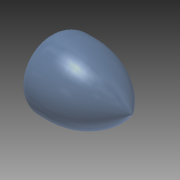
# Autodesk Inventor part: eye
Saved by Autodesk Inventor 2015 (Build 190159000, 159)
## iProperties
Created: 2015-03-17
Part Number: eye
Material: Genérico
Document SubType Name: Modeling
Designer: david_000
Density: 1 g/cm^3
Appearance: Valor por defecto
Author: david_000
Autodesk Inventor part; units mm, degrees
ref_plane "YZ Plane" through (0, 0, 0) normal (1, 0, 0) x (0, 1, 0)
ref_plane "XZ Plane" through (0, 0, 0) normal (0, 1, 0) x (-1, 0, 0)
ref_plane "XY Plane" through (0, 0, 0) normal (0, 0, 1) x (1, 0, 0)
sketch "Boceto1" plane through (0, 0, 0) normal (0, 1, 0) x (-1, 0, 0)
  line L0 (135, 0) -> (135, 20)
  line L1 (135, 20) -> (135, 65)
  line L2 (135, 65) -> (35, 65)
  line L3 (135, 0) -> (92.5, 0)
  line L4 (135, 20) -> (115, 20)
  arc A0 (35, 65) -> (115, 20) centre (115, 113.6111) ccw
  line L5 (40.5241, 62) -> (132, 62)
  line L6 (132, 62) -> (132, 23)
  line L7 (135, 23) -> (115, 23)
  arc A1 (38.5321, 65) -> (115, 23) centre (115, 113.6111) ccw
  line L8 (135, 0) -> (135, -20)
  line L9 (135, -20) -> (135, -65)
  line L10 (135, -65) -> (35, -65)
  line L11 (135, -20) -> (115, -20)
  arc A2 (115, -20) -> (35, -65) centre (115, -113.6111) ccw
  line L12 (40.5241, -62) -> (132, -62)
  line L13 (132, -62) -> (132, -23)
  line L14 (135, -23) -> (115, -23)
  arc A3 (115, -23) -> (38.5321, -65) centre (115, -113.6111) ccw
  point P0 (0, 0)
  point P1 (0, 0)
  dimension "d0" = 20
  dimension "d1" = 45
  dimension "d2" = 20
  dimension "d3" = 100
  dimension "d4" = 90
  dimension "d5" = 20
  dimension "d6" = 135
  dimension "d7" = 3
  constraints: 30 end point, 11 symmetric about line, 10 point on circle, 8 point on line, 4 centre point, 4 perpendicular, 1 horizontal, 1 tangent, 1 vertical, 3 other
  measures "d0" distance of L0.start L0.end
  measures "d1" distance of L0.end L1.end
  measures "d2" distance of L0.end L4.end
  measures "d3" distance of L1.end L2.end
  measures "d4" angle of L2 L1
  measures "d5" vertical distance of L0.end point (0, 0)
  measures "d6" horizontal distance of point (0, 0) L1.end
  measures "d7" distance between parallel lines of L2 L5
revolve "Revolución1" add sketch "Boceto1" angle 360 about axis through (-135, 0, -65) along (1, 0, 0) contours L9 L10 A3 L12 L13 L14 | L13 L12 A3 L14
sketch "Boceto3" plane through (-135, 0, -65) normal (-1, 0, 0) x (0, 0, 1)
  circle A0 centre (0, 0) radius 42
  point P0 (65, 0)
  constraints: 1 centre point
extrude "Extrusión2" add sketch "Boceto3" along normal blind 10
fillet "Empalme3" radius 20 1 edges at (-145, 0, -107)
